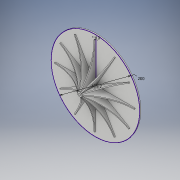
# Autodesk Inventor part: TurntablePlatform
Saved by Autodesk Inventor 2019.3 (Build 233278000, 278)
## iProperties
Created: 2019-07-08
Part Number: TurntablePlatform
Material: Generic
Document SubType Name: Modeling
Designer: mark
Density: 1 g/cm^3
Appearance: Default
Author: mark
Autodesk Inventor part; units mm, degrees
ref_plane "YZ Plane" through (0, 0, 0) normal (1, 0, 0) x (0, 1, 0)
ref_plane "XZ Plane" through (0, 0, 0) normal (0, 1, 0) x (-1, 0, 0)
ref_plane "XY Plane" through (0, 0, 0) normal (0, 0, 1) x (1, 0, 0)
sketch "Sketch1" plane through (0, 0, 0) normal (0, 0, 1) x (1, 0, 0)
  circle A0 centre (0, 0) radius 2.6
  circle A1 centre (0, 0) radius 100
  line L0 (-1, 90) -> (1, 90)
  line L1 (1, 90) -> (1, 2.4)
  line L2 (1, 2.4) -> (-1, 2.4)
  line L3 (-1, 2.4) -> (-1, 90)
  dimension "d0" = 5.2
  dimension "d1" = 200
  dimension "d2" = 2
  dimension "d3" = 1
  dimension "d4" = 10
  constraints: 8 end point, 2 centre point, 2 coincident, 2 point on circle, 1 horizontal, 1 vertical
  measures "d0" diameter of A0
  measures "d1" diameter of A1
  measures "d2" distance between parallel lines of L1 L3
  measures "d3" distance from line of L3 point (0, 0)
  measures "d4" distance edge to line of A1 L0
extrude "Extrusion1" add sketch "Sketch1" against normal blind 3 contours A0 L2 | A0 L3 L0 L1 | A1 picked at (-0.1543, 0.6409)
extrude "Extrusion2" add sketch "Sketch1" along normal blind 35 contours A0 L3 L0 L1
sketch "Sketch2" plane through (-1, 2.4, 0) normal (-1, 0, 0) x (0, 0, 1)
  line L0 (0, 87.6) -> (35, 87.6) projected
  arc A0 (2, 87.6) -> (35, 2) centre (129.5206, 87.6) ccw
  line L1 (0, 97.6) -> (0, -102.4) projected
  line L2 (0, 0) -> (35, 0) projected
  line L3 (35, 87.6) -> (35, 0) projected
  line L4 (0, 87.6) -> (35, 87.6) projected
  point P0 (0, -2.4)
  dimension "d9" = 2
  dimension "d10" = 2
  constraints: 3 point on line, 2 point on circle, 1 centre point
  measures "d9" distance from line of A0.start L1
  measures "d10" distance from line of L2 A0.end
extrude "Extrusion3" cut sketch "Sketch2" against normal up to next contours L0 L3 A0
pattern_circular "Circular Pattern1" count 12 over 360 about axis through (0, 0, 0) along (0, 0, 1) of "Extrusion3", "Extrusion2"
sketch "Sketch3" plane through (0, 0, 35) normal (0, 0, 1) x (1, 0, 0)
  circle A0 centre (0, 0) radius 5
  arc A1 (2.2, 2.0396) -> (2.2, -2.0396) centre (0, 0) ccw
  line L0 (2.2, 2.0396) -> (2.2, -2.0396)
  dimension "d19" = 10
  dimension "d22" = 3
  dimension "d23" = 2.2
  constraints: 2 centre point, 2 coincident, 2 end point, 2 point on circle, 1 vertical
  measures "d19" diameter of A0
  measures "d22" radius of A1
  measures "d23" distance from line of A1.centre L0
extrude "Extrusion4" add sketch "Sketch3" against normal up to next
body "Solid1"
